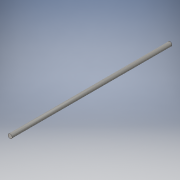
# Autodesk Inventor part: 98848A011
Saved by Autodesk Inventor 2016 SP1 (Build 200210100, 210)
## iProperties
Created: 2017-02-16
Part Number: 98848A011
Material: Stainless Steel
Document SubType Name: Modeling
Designer: 601898
Density: 8 g/cm^3
Appearance: Semi-Polished
Description: 10-32 Stainless Steel Threaded Rod
Author: 601898
Title: 98848A011
Autodesk Inventor part; units mm, degrees
ref_plane "YZ Plane" through (0, 0, 0) normal (1, 0, 0) x (0, 1, 0)
ref_plane "XZ Plane" through (0, 0, 0) normal (0, 1, 0) x (-1, 0, 0)
ref_plane "XY Plane" through (0, 0, 0) normal (0, 0, 1) x (1, 0, 0)
sketch "Sketch1" plane through (0, 0, 0) normal (0, 0, 1) x (1, 0, 0)
  circle A0 centre (0, 0) radius 3.9688
  dimension "d0" = 7.9375
  constraints: 1 centre point, 1 coincident
  measures "d0" diameter of A0
extrude "Extrusion1" add sketch "Sketch1" along normal blind 304.8
thread "Thread1" size "5/16-18 UNC" class "2A" standard "ANSI Unified Screw Threads" full length
body "Solid1"
